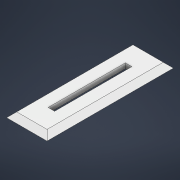
# Autodesk Inventor part: HornHolder
Saved by Autodesk Inventor 2022 (Build 260153000, 153)
## iProperties
Created: 2022-06-02
Part Number: HornHolder
Material: ABS プラスチック
Document SubType Name: Modeling
Designer: neko2
Density: 1.06 g/cm^3
Appearance: 滑らか - 白
Mass: 0.15735 g
Surface Area: 4.19101 cm^2
Volume: 0.148443 cm^3
Author: neko2
Autodesk Inventor part; units mm, degrees
ref_plane "YZ Plane" through (0, 0, 0) normal (1, 0, 0) x (0, 1, 0)
ref_plane "XZ Plane" through (0, 0, 0) normal (0, 1, 0) x (-1, 0, 0)
ref_plane "XY Plane" through (0, 0, 0) normal (0, 0, 1) x (1, 0, 0)
sketch "スケッチ1" plane through (0, 0, 0) normal (0, 1, 0) x (-1, 0, 0)
  line L0 (-0.65, 7.65) -> (0.65, 7.65)
  line L1 (0.65, 7.65) -> (0.65, -7.65)
  line L2 (0.65, -7.65) -> (-0.65, -7.65)
  line L3 (-0.65, -7.65) -> (-0.65, 7.65)
  line L4 (-0.65, 7.65) -> (0.65, -7.65) construction
  line L5 (0.65, 7.65) -> (-0.65, -7.65) construction
  line L6 (-4, 12.5) -> (4, 12.5)
  line L7 (4, 12.5) -> (4, -12.5)
  line L8 (4, -12.5) -> (-4, -12.5)
  line L9 (-4, -12.5) -> (-4, 12.5)
  line L10 (-4, 12.5) -> (4, -12.5) construction
  line L11 (4, 12.5) -> (-4, -12.5) construction
  point P0 (0, 0)
  dimension "d0" = 1.3
  dimension "d1" = 15.3
  dimension "d2" = 8
  dimension "d3" = 25
  constraints: 24 end point, 4 midpoint, 4 parallel, 2 horizontal, 2 perpendicular
  measures "d0" distance of L1.end L2.end
  measures "d1" distance of L0.end L1.end
  measures "d2" distance of L7.end L8.end
  measures "d3" distance of L6.end L7.end
extrude "押し出し1" add sketch "スケッチ1" along normal blind 1
chamfer "面取り1" distance 1 angle 45 4 edges at (-4, 1, 0) (0, 1, -12.5) (4, 1, 0) (0, 1, 12.5)
